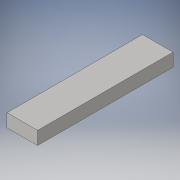
# Autodesk Inventor part: 2x4 17.5 Inch
Saved by Autodesk Inventor 2016 (Build 200138000, 138)
## iProperties
Created: 2015-07-07
Part Number: 2x4 17.5 Inch
Material: Generic
Document SubType Name: Modeling
Designer: steele
Density: 1 g/cm^3
Appearance: Default
Author: steele
Autodesk Inventor part; units mm, degrees
ref_plane "YZ Plane" through (0, 0, 0) normal (1, 0, 0) x (0, 1, 0)
ref_plane "XZ Plane" through (0, 0, 0) normal (0, 1, 0) x (-1, 0, 0)
ref_plane "XY Plane" through (0, 0, 0) normal (0, 0, 1) x (1, 0, 0)
sketch "Sketch1" plane through (0, 0, 0) normal (0, 1, 0) x (-1, 0, 0)
  line L0 (-44.45, 196.85) -> (-44.45, -196.85)
  line L1 (-44.45, -196.85) -> (44.45, -196.85)
  line L2 (44.45, -196.85) -> (44.45, 196.85)
  line L3 (44.45, 196.85) -> (-44.45, 196.85)
  line L4 (-44.45, 196.85) -> (44.45, -196.85) construction
  line L5 (-44.45, -196.85) -> (44.45, 196.85) construction
  point P0 (0, 0)
  dimension "d0" = 88.9
  dimension "length" = 393.7
  constraints: 12 end point, 2 midpoint, 2 parallel, 1 perpendicular, 1 vertical
  measures "d0" distance of L2.end L0.start
  measures "length" distance of L1.end L2.end
extrude "Extrusion1" add sketch "Sketch1" along normal blind 38.1
body "Solid1"
